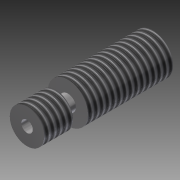
# Autodesk Inventor part: E3DV6HeatBreak
Saved by Autodesk Inventor 2015 (Build 190159000, 159)
## iProperties
Created: 2014-08-17
Part Number: E3DV6HeatBreak
Material: Stainless Steel
Document SubType Name: Modeling
Designer: Jack
Density: 8 g/cm^3
Appearance: Semi-Polished
Author: Jack
Autodesk Inventor part; units mm, degrees
ref_plane "YZ Plane" through (0, 0, 0) normal (1, 0, 0) x (0, 1, 0)
ref_plane "XZ Plane" through (0, 0, 0) normal (0, 1, 0) x (-1, 0, 0)
ref_plane "XY Plane" through (0, 0, 0) normal (0, 0, 1) x (1, 0, 0)
sketch "Sketch1" plane through (0, 0, 0) normal (0, 0, 1) x (1, 0, 0)
  line L0 (0, 0) -> (3, 0)
  line L1 (3, 0) -> (3, 5)
  line L2 (3, 5) -> (1.4, 5)
  line L3 (1.4, 5) -> (1.4, 7.1)
  line L4 (1.4, 7.1) -> (3.5, 7.1)
  line L5 (3.5, 7.1) -> (3.5, 21.9)
  line L6 (3.5, 21.9) -> (0, 21.9)
  line L7 (0, 21.9) -> (0, 0)
  dimension "d0" = 3
  dimension "d1" = 5
  dimension "d2" = 1.4
  dimension "d3" = 2.1
  dimension "d4" = 3.5
  dimension "d5" = 14.8
  constraints: 16 end point, 5 perpendicular, 2 vertical, 1 horizontal
  measures "d0" distance of L0.start L0.end
  measures "d1" distance of L0.end L1.end
  measures "d2" horizontal distance of L0.start L2.end
  measures "d3" distance of L2.end L3.end
  measures "d4" horizontal distance of L0.start L4.end
  measures "d5" distance of L4.end L5.end
revolve "Revolution1" add sketch "Sketch1" angle 360 about axis through (0, 21.9, 0) along (0, -1, 0)
thread "Thread1" size "M6x1" class "6g" standard "ANSI Metric M Profile" full length
thread "Thread2" size "M7x1" class "6g" standard "ANSI Metric M Profile" full length
sketch "Sketch2" plane through (0, 0, 0) normal (0, -1, 0) x (1, 0, 0)
  circle A0 centre (0, 0) radius 3.5 projected
  circle A1 centre (0, 0) radius 1
  dimension "d11" = 2
  constraints: 1 centre point, 1 coincident
  measures "d11" diameter of A1
extrude "Extrusion1" cut sketch "Sketch2" against normal up to surface (21.9 mm away) contours A1
sketch "Sketch3" plane through (0, 21.9, 0) normal (0, 1, 0) x (1, 0, 0)
  circle A0 centre (0, 0) radius 1 projected
  circle A1 centre (0, 0) radius 3.5 projected
  circle A2 centre (0, 0) radius 2.1
  dimension "d14" = 4.2
  constraints: 1 centre point, 1 coincident
  measures "d14" diameter of A2
extrude "Extrusion2" cut sketch "Sketch3" against normal blind 10.5 contours A2
body "Solid1"
